Solar_Panel_Fit (Autodesk Fusion 360 design; units mm, degrees)
part number: 2026-09-24-14-30-26-043
Autodesk Fusion 360 part; units mm, degrees
sketch "Sketch1" plane through (0, 0, 0) normal (0, 0, 1) x (1, 0, 0)
  line L0 (0, 0) -> (145, 0)
  line L1 (145, 0) -> (145, -145)
  line L2 (145, -145) -> (0, -145)
  line L3 (0, -145) -> (0, 0)
  dimension "d1" = 145
  dimension "d2" = 145
  constraint horizontal L0
  constraint vertical L1
  constraint horizontal L2
  constraint vertical L3
  constraint coincident L0.start L3.end
  measures "d1" distance of L0.start L0.end
  measures "d2" distance of L0.start L2.end
extrude "Extrude1" add sketch "Sketch1" along normal blind 5 makes body 1
sketch "Sketch2" plane through (0, 0, 5) normal (0, 0, 1) x (-1, 0, 0)
  line L0 (0, 145) -> (-145, 145)
  line L1 (-145, 145) -> (-145, 0)
  line L2 (-145, 0) -> (0, 0)
  line L3 (0, 0) -> (0, 145)
  line L4 (-145, 145) -> (0, 145)
  line L5 (0, 145) -> (0, 0)
  line L6 (0, 0) -> (-145, 0)
  line L7 (-145, 0) -> (-145, 145)
  constraint horizontal L4
  constraint vertical L5
  constraint horizontal L6
  constraint vertical L7
  constraint coincident L2.end L3.start
  constraint coincident L0.end L1.start
extrude "Extrude2" add 1 faces at (48.3333, 0, 3.3333) along direction (0, 1, 0) blind 5 on bodies 1 bodies 1
extrude "Extrude3" add 1 faces at (145, -45, 1.6667) along direction (1, 0, 0) blind 5 on bodies 1 bodies 1
extrude "Extrude4" add 1 faces at (100, -145, 3.3333) along direction (0, -1, 0) blind 5 on bodies 1 bodies 1
extrude "Extrude5" add 1 faces at (0, -46.6667, 1.6667) along direction (-1, 0, 0) blind 5 on bodies 1 bodies 1
extrude "Extrude6" add sketch "Sketch2" along normal blind 5 bodies 1
extrude "Extrude7" add 1 faces at (96.6667, -96.6667, 10) along direction (0, 0, 1) blind 1 on bodies 1 bodies 1
extrude "Extrude8" add 1 faces at (96.6667, 3.3333, 5) along direction (0, 0, 1) blind 5 on bodies 1 bodies 1
extrude "Extrude9" cut 1 faces at (96.6667, -96.6667, 11) along direction (0, 0, -1) blind 6 on bodies 1 bodies 1
move_face "OffsetFaces1" offset -0.15 1 faces at (96.6667, 0, 6.6667) on bodies 1
extrude "Extrude10" cut 1 faces at (145, -96.6167, 8.3333) along direction (1, 0, 0) blind 0.15 on bodies 1 bodies 1
extrude "Extrude11" cut 1 faces at (48.3833, -145, 8.3333) along direction (0, -1, 0) blind 0.15 on bodies 1 bodies 1
extrude "Extrude12" cut 1 faces at (0, -48.2833, 8.3333) along direction (-1, 0, 0) blind 0.15 on bodies 1 bodies 1
extrude "Extrude13" add 1 faces at (46.6667, 5, 3.3333) along direction (0, 1, 0) blind 5 on bodies 1 bodies 1
extrude "Extrude14" add 1 faces at (-5, -43.3333, 3.3333) along direction (-1, 0, 0) blind 5 on bodies 1 bodies 1
extrude "Extrude15" add 1 faces at (150, -43.3333, 3.3333) along direction (1, 0, 0) blind 5 on bodies 1 bodies 1
extrude "Extrude16" add 1 faces at (100, -150, 3.3333) along direction (0, -1, 0) blind 5 on bodies 1 bodies 1
sketch "Sketch3" plane through (0, 0, 10) normal (0, 0, 1) x (-1, 0, 0)
  line L0 (0.15, -0.15) -> (-145.15, -0.15)
  line L1 (-145.15, -0.15) -> (-145.15, 145.15)
  line L2 (-145.15, 145.15) -> (0.15, 145.15)
  line L3 (0.15, 145.15) -> (0.15, -0.15)
  line L4 (-155, -10) -> (10, -10)
  line L5 (10, -10) -> (10, 155)
  line L6 (10, 155) -> (-155, 155)
  line L7 (-155, 155) -> (-155, -10)
  line L8 (10, -10) -> (10, 72.5) construction
  line L9 (10, 72.5) -> (0.15, 72.5) construction
  line L10 (0.15, 72.5) -> (0.15, 57.5) construction
  line L11 (0.15, 72.5) -> (0.15, 87.5) construction
  line L12 (0.15, 72.5) -> (0.15, 67.5) construction
  line L13 (0.15, 72.5) -> (0.15, 77.5) construction
  line L14 (0.15, 77.5) -> (10, 77.5) construction
  line L15 (10, 77.5) -> (5.075, 77.5) construction
  line L16 (0.15, 57.5) -> (5.075, 57.5) construction
  line L17 (0.15, 57.5) -> (2.6125, 57.5) construction
  line L18 (2.5, 57.5) -> (5.075, 57.5)
  line L19 (5.075, 57.5) -> (5.075, 87.5)
  line L20 (5.075, 87.5) -> (2.5, 87.5)
  line L21 (2.5, 87.5) -> (2.5, 57.5)
  dimension "d36" = 15
  dimension "d37" = 15
  dimension "d38" = 5
  dimension "d39" = 5
  dimension "d40" = 4.925
  constraint coincident L4.end L5.start
  constraint midpoint L5 L8.end
  constraint midpoint L3 L9.end
  constraint perpendicular L9 L10
  constraint perpendicular L9 L11
  constraint perpendicular L9 L12
  constraint perpendicular L9 L13
  constraint coincident L5 L14.end
  constraint perpendicular L5 L14
  constraint midpoint L14 L15.end
  constraint horizontal L16
  constraint midpoint L16 L17.end
  constraint horizontal L18
  constraint vertical L19
  constraint horizontal L20
  constraint vertical L21
  constraint coincident L16 L18.start
  measures "d36" distance of L9.end L10.end
  measures "d37" distance of L9.end L11.end
  measures "d38" distance of L9.end L12.end
  measures "d39" distance of L9.end L13.end
  measures "d40" distance of L10.end L16.end
extrude "Extrude17" cut sketch "Sketch3" against normal blind 5 contours L18 L19 L20 L21 bodies 1
sketch "Sketch4" plane through (0, 0, 10) normal (0, 0, 1) x (-1, 0, 0)
  line L0 (5.075, 57.5) -> (2.5, 57.5)
  line L1 (2.5, 57.5) -> (2.5, 87.5)
  line L2 (2.5, 87.5) -> (5.075, 87.5)
  line L3 (5.075, 87.5) -> (5.075, 57.5)
  line L4 (0.15, -0.15) -> (-145.15, -0.15)
  line L5 (-145.15, -0.15) -> (-145.15, 145.15)
  line L6 (-145.15, 145.15) -> (0.15, 145.15)
  line L7 (0.15, 145.15) -> (0.15, -0.15)
  line L8 (-155, -10) -> (10, -10)
  line L9 (10, -10) -> (10, 155)
  line L10 (10, 155) -> (-155, 155)
  line L11 (-155, 155) -> (-155, -10)
  line L12 (2.5, 57.5) -> (2.5, 87.5) construction
  line L13 (2.5, 87.5) -> (2.5, 72.5) construction
  line L14 (2.5, 72.5) -> (2.5, 80) construction
  line L15 (2.5, 72.5) -> (2.5, 57.5) construction
  line L16 (2.5, 57.5) -> (2.5, 65) construction
  line L17 (2.5, 65.1) -> (2.5, 80)
  line L18 (2.5, 80) -> (0.15, 80)
  line L19 (0.15, 80) -> (0.15, 65)
  line L20 (0.15, 65) -> (2.5, 65)
  line L21 (2.5, 65) -> (2.5, 80)
  constraint coincident L0.end L1.start
  constraint coincident L1.end L2.start
  constraint midpoint L12 L13.end
  constraint midpoint L13 L14.end
  constraint midpoint L15 L16.end
  constraint coincident L15 L17.start
  constraint horizontal L18
  constraint vertical L19
  constraint horizontal L20
  constraint vertical L21
  constraint coincident L7 L19.end
extrude "Extrude18" cut sketch "Sketch4" against normal blind 5 contours L1 L7 L17 L18 L19 L20 L21 bodies 1
sketch "Sketch5" plane through (0, 0, 10) normal (0, 0, 1) x (-1, 0, 0)
  line L0 (-155, -10) -> (10, -10)
  line L1 (10, -10) -> (10, 155)
  line L2 (10, 155) -> (-155, 155)
  line L3 (-155, 155) -> (-155, -10)
  line L4 (0.15, 80) -> (2.5, 80)
  line L5 (2.5, 80) -> (2.5, 87.5)
  line L6 (2.5, 87.5) -> (5.075, 87.5)
  line L7 (5.075, 87.5) -> (5.075, 57.5)
  line L8 (5.075, 57.5) -> (2.5, 57.5)
  line L9 (2.5, 57.5) -> (2.5, 65)
  line L10 (2.5, 65) -> (0.15, 65)
  line L11 (0.15, 65) -> (0.15, -0.15)
  line L12 (0.15, -0.15) -> (-145.15, -0.15)
  line L13 (-145.15, -0.15) -> (-145.15, 145.15)
  line L14 (-145.15, 145.15) -> (0.15, 145.15)
  line L15 (0.15, 145.15) -> (0.15, 80)
  line L16 (2.5, 57.5) -> (2.5, 65)
  line L17 (2.5, 65) -> (0.15, 65)
  line L18 (5.075, 57.5) -> (2.5, 57.5)
  line L19 (5.075, 87.5) -> (5.075, 57.5)
  line L20 (2.5, 87.5) -> (5.075, 87.5)
  line L21 (0.15, 80) -> (2.5, 80)
  line L22 (2.5, 80) -> (2.5, 87.5)
  line L23 (0.15, 80) -> (0.15, 65)
  line L24 (5.075, 57.5) -> (2.5, 57.5)
  line L25 (2.5, 57.5) -> (2.5, 65)
  line L26 (2.5, 65) -> (0.15, 65)
  line L27 (5.075, 57.5) -> (5.075, 87.5)
  line L28 (2.5, 87.5) -> (5.075, 87.5)
  line L29 (2.5, 87.5) -> (2.5, 80)
  line L30 (2.5, 80) -> (0.15, 80)
  line L31 (0.15, 80) -> (0.15, 65)
  constraint coincident L4.start L15.end
  constraint coincident L10.end L11.start
  constraint coincident L7.end L8.start
  constraint coincident L8.end L9.start
  constraint coincident L9.end L10.start
  constraint coincident L6.end L7.start
  constraint coincident L5.end L6.start
  constraint coincident L4.end L5.start
  constraint perpendicular L15 L30
extrude "Extrude19" add sketch "Sketch5" along normal blind 1 separate body contours L4 L5 L6 L7 L8 L9 L10 L16 L17 L18 L19 L20 L21 L22 L23 L24 L25 L26 L27 L28 L29 L30 L31 makes body 2
move_body "Move1" bodies 2 to x (-1, 0, 0) y (0, -1, 0) z (0, 0, 1) at (144.775, -145, 0)
copy_body "CopyPasteBodies1" bodies 2 makes body 3
move_body "Move2" bodies 3 to x (0, 1, 0) y (-1, 0, 0) z (0, 0, 1) at (-0.1125, -144.8875, 0)
copy_body "CopyPasteBodies2" bodies 3 makes body 4
move_body "Move3" bodies 4 to x (-1, 0, 0) y (0, -1, 0) z (0, 0, 1) at (144.775, -145, 0)
extrude "Extrude20" cut 3 faces at (148.9917, -75, 11) (74.8875, -149.1042, 11) (74.8875, 4.1042, 11) along direction (0, 0, -1) blind 6 on bodies 2 3 4 bodies 1 2 3 4
extrude "Extrude21" cut 1 faces at (148.1333, -57.5, 8.3333) along direction (0, 1, 0) blind 5 on bodies 1 bodies 1
extrude "Extrude22" cut 1 faces at (148.9917, -87.5, 8.3333) along direction (0, -1, 0) blind 5 on bodies 1 bodies 1
extrude "Extrude23" cut 1 faces at (87.3875, 4.1042, 8.3333) along direction (1, 0, 0) blind 5 on bodies 1 bodies 1
extrude "Extrude24" cut 1 faces at (57.3875, 3.2458, 8.3333) along direction (-1, 0, 0) blind 5 on bodies 1 bodies 1
extrude "Extrude25" cut 1 faces at (-4.2167, -87.5, 8.3333) along direction (0, -1, 0) blind 5 on bodies 1 bodies 1
extrude "Extrude26" cut 1 faces at (-3.3583, -57.5, 8.3333) along direction (0, 1, 0) blind 5 on bodies 1 bodies 1
extrude "Extrude27" cut 1 faces at (57.3875, -149.1042, 8.3333) along direction (-1, 0, 0) blind 5 on bodies 1 bodies 1
extrude "Extrude28" cut 1 faces at (87.3875, -148.2458, 8.3333) along direction (1, 0, 0) blind 5 on bodies 1 bodies 1
extrude "Extrude29" cut 1 faces at (52.3875, -149.1042, 8.3333) along direction (-1, 0, 0) blind 2.5 on bodies 1 bodies 1
extrude "Extrude30" cut 1 faces at (92.3875, -148.2458, 8.3333) along direction (1, 0, 0) blind 2.5 on bodies 1 bodies 1
extrude "Extrude31" cut 1 faces at (-4.2167, -92.5, 8.3333) along direction (0, -1, 0) blind 2.5 on bodies 1 bodies 1
extrude "Extrude32" cut 1 faces at (-3.3583, -52.5, 8.3333) along direction (0, 1, 0) blind 2.5 on bodies 1 bodies 1
extrude "Extrude33" cut 1 faces at (52.3875, 3.2458, 8.3333) along direction (-1, 0, 0) blind 2.5 on bodies 1 bodies 1
extrude "Extrude34" cut 1 faces at (92.3875, 4.1042, 8.3333) along direction (1, 0, 0) blind 2.5 on bodies 1 bodies 1
extrude "Extrude35" cut 1 faces at (148.1333, -52.5, 8.3333) along direction (0, 1, 0) blind 2.5 on bodies 1 bodies 1
extrude "Extrude36" cut 1 faces at (148.9917, -92.5, 8.3333) along direction (0, -1, 0) blind 2.5 on bodies 1 bodies 1
extrude "Extrude37" add 1 faces at (53.2083, -70, 5) along direction (0, 0, 1) blind 2.5 on bodies 1 bodies 1 2 3 4
sketch "Sketch6" plane through (0, 0, 10) normal (0, 0, 1) x (-1, 0, 0)
  line L0 (-149.85, 50) -> (-149.85, 95)
  line L1 (-149.85, 95) -> (-147.275, 95)
  line L2 (-147.275, 95) -> (-147.275, 80)
  line L3 (-147.275, 80) -> (-145.15, 80)
  line L4 (-145.15, 80) -> (-145.15, 145.15)
  line L5 (-145.15, 145.15) -> (-79.8875, 145.15)
  line L6 (-79.8875, 145.15) -> (-79.8875, 147.3875)
  line L7 (-79.8875, 147.3875) -> (-94.8875, 147.3875)
  line L8 (-94.8875, 147.3875) -> (-94.8875, 149.9625)
  line L9 (-94.8875, 149.9625) -> (-49.8875, 149.9625)
  line L10 (-49.8875, 149.9625) -> (-49.8875, 147.3875)
  line L11 (-49.8875, 147.3875) -> (-64.8875, 147.3875)
  line L12 (-64.8875, 147.3875) -> (-64.8875, 145.15)
  line L13 (-64.8875, 145.15) -> (0.15, 145.15)
  line L14 (0.15, 145.15) -> (0.15, 80)
  line L15 (0.15, 80) -> (2.5, 80)
  line L16 (2.5, 80) -> (2.5, 95)
  line L17 (2.5, 95) -> (5.075, 95)
  line L18 (5.075, 95) -> (5.075, 50)
  line L19 (5.075, 50) -> (2.5, 50)
  line L20 (2.5, 50) -> (2.5, 65)
  line L21 (2.5, 65) -> (0.15, 65)
  line L22 (0.15, 65) -> (0.15, -0.15)
  line L23 (0.15, -0.15) -> (-64.8875, -0.15)
  line L24 (-64.8875, -0.15) -> (-64.8875, -2.3875)
  line L25 (-64.8875, -2.3875) -> (-49.8875, -2.3875)
  line L26 (-49.8875, -2.3875) -> (-49.8875, -4.9625)
  line L27 (-49.8875, -4.9625) -> (-94.8875, -4.9625)
  line L28 (-94.8875, -4.9625) -> (-94.8875, -2.3875)
  line L29 (-94.8875, -2.3875) -> (-79.8875, -2.3875)
  line L30 (-79.8875, -2.3875) -> (-79.8875, -0.15)
  line L31 (-79.8875, -0.15) -> (-145.15, -0.15)
  line L32 (-145.15, -0.15) -> (-145.15, 65)
  line L33 (-145.15, 65) -> (-147.275, 65)
  line L34 (-147.275, 65) -> (-147.275, 50)
  line L35 (-147.275, 50) -> (-149.85, 50)
  line L36 (-155, -10) -> (10, -10)
  line L37 (10, -10) -> (10, 155)
  line L38 (10, 155) -> (-155, 155)
  line L39 (-155, 155) -> (-155, -10)
  line L40 (0.15, 145.15) -> (0.15, 95) construction
  line L41 (0.15, 95) -> (0.15, 120.075) construction
  circle A0 centre (0.15, 120.075) radius 5
  dimension "d83" = 10
  constraint coincident L13.end L14.start
  constraint coincident L14 L40.end
  constraint midpoint L40 L41.end
  constraint coincident L41.end A0.centre
  measures "d83" diameter of A0
extrude "Extrude38" cut sketch "Sketch6" against normal blind 2.5 contours L14 A0 picked at (1.5521, 119.1739) bodies 1
extrude "Extrude39" add 1 faces at (100, -45, 0) along direction (0, 0, -1) blind 5 on bodies 1 bodies 1
move_body "Move4" bodies 1 to x (1, 0, 0) y (0, 1, 0) z (0, 0, 1) at (0, 0, 5)
sketch "Sketch7" plane through (0, 0, 12.5) normal (0, 0, 1) x (-1, 0, 0)
  line L0 (-79.8875, 145.15) -> (-145.15, 145.15)
  line L1 (-145.15, 145.15) -> (-145.15, 80)
  line L2 (-145.15, 80) -> (-147.275, 80)
  line L3 (-147.275, 80) -> (-147.275, 95)
  line L4 (-147.275, 95) -> (-149.85, 95)
  line L5 (-149.85, 95) -> (-149.85, 50)
  line L6 (-149.85, 50) -> (-147.275, 50)
  line L7 (-147.275, 50) -> (-147.275, 65)
  line L8 (-147.275, 65) -> (-145.15, 65)
  line L9 (-145.15, 65) -> (-145.15, -0.15)
  line L10 (-145.15, -0.15) -> (-79.8875, -0.15)
  line L11 (-79.8875, -0.15) -> (-79.8875, -2.3875)
  line L12 (-79.8875, -2.3875) -> (-94.8875, -2.3875)
  line L13 (-94.8875, -2.3875) -> (-94.8875, -4.9625)
  line L14 (-94.8875, -4.9625) -> (-49.8875, -4.9625)
  line L15 (-49.8875, -4.9625) -> (-49.8875, -2.3875)
  line L16 (-49.8875, -2.3875) -> (-64.8875, -2.3875)
  line L17 (-64.8875, -2.3875) -> (-64.8875, -0.15)
  line L18 (-64.8875, -0.15) -> (0.15, -0.15)
  line L19 (0.15, -0.15) -> (0.15, 65)
  line L20 (0.15, 65) -> (2.5, 65)
  line L21 (2.5, 65) -> (2.5, 50)
  line L22 (2.5, 50) -> (5.075, 50)
  line L23 (5.075, 50) -> (5.075, 95)
  line L24 (5.075, 95) -> (2.5, 95)
  line L25 (2.5, 95) -> (2.5, 80)
  line L26 (2.5, 80) -> (0.15, 80)
  line L27 (0.15, 80) -> (0.15, 115.075)
  arc A0 (0.15, 115.075) -> (0.15, 125.075) centre (0.15, 120.075) ccw
  line L28 (0.15, 125.075) -> (0.15, 145.15)
  line L29 (0.15, 145.15) -> (-64.8875, 145.15)
  line L30 (-64.8875, 145.15) -> (-64.8875, 147.3875)
  line L31 (-64.8875, 147.3875) -> (-49.8875, 147.3875)
  line L32 (-49.8875, 147.3875) -> (-49.8875, 149.9625)
  line L33 (-49.8875, 149.9625) -> (-94.8875, 149.9625)
  line L34 (-94.8875, 149.9625) -> (-94.8875, 147.3875)
  line L35 (-94.8875, 147.3875) -> (-79.8875, 147.3875)
  line L36 (-79.8875, 147.3875) -> (-79.8875, 145.15)
  line L37 (10, 155) -> (-155, 155) construction
  line L38 (-155, 155) -> (-72.5, 155) construction
  line L39 (-72.5, 155) -> (-72.3875, 149.9625) construction
  line L40 (-72.3875, 149.9625) -> (-72.3875, 137.4625) construction
  line L41 (-72.3875, 137.4625) -> (-97.3875, 137.4625) construction
  line L42 (-72.3875, 137.4625) -> (-47.3875, 137.4625) construction
  line L43 (-72.3875, 137.4625) -> (-72.3875, 92.4625) construction
  line L44 (-72.3875, 92.4625) -> (-47.3875, 92.4625) construction
  line L45 (-47.3875, 92.4625) -> (-97.3875, 92.4625)
  line L46 (-97.3875, 92.4625) -> (-97.3875, 137.4625)
  line L47 (-97.3875, 137.4625) -> (-47.3875, 137.4625)
  line L48 (-47.3875, 137.4625) -> (-47.3875, 92.4625)
  dimension "d88" = 12.5
  dimension "d89" = 25
  dimension "d90" = 25
  dimension "d91" = 45
  constraint perpendicular L28 L37
  constraint midpoint L37 L38.end
  constraint midpoint L33 L39.end
  constraint perpendicular L33 L40
  constraint perpendicular L40 L41
  constraint perpendicular L40 L42
  constraint perpendicular L42 L43
  constraint perpendicular L43 L44
  constraint horizontal L45
  constraint vertical L46
  constraint horizontal L47
  constraint vertical L48
  measures "d88" distance of L39.end L40.end
  measures "d89" distance of L40.end L41.end
  measures "d90" distance of L40.end L42.end
  measures "d91" distance of L40.end L43.end
extrude "Extrude40" cut sketch "Sketch7" against normal blind 70 contours L45 L46 L47 L48 bodies 1
sketch "Sketch8" plane through (0, 0, 12.5) normal (0, 0, 1) x (-1, 0, 0)
  line L0 (-97.3875, 92.4625) -> (-97.3875, 137.4625)
  line L1 (-97.3875, 137.4625) -> (-47.3875, 137.4625)
  line L2 (-47.3875, 137.4625) -> (-47.3875, 92.4625)
  line L3 (-47.3875, 92.4625) -> (-97.3875, 92.4625)
  line L4 (-79.8875, 145.15) -> (-145.15, 145.15)
  line L5 (-145.15, 145.15) -> (-145.15, 80)
  line L6 (-145.15, 80) -> (-147.275, 80)
  line L7 (-147.275, 80) -> (-147.275, 95)
  line L8 (-147.275, 95) -> (-149.85, 95)
  line L9 (-149.85, 95) -> (-149.85, 50)
  line L10 (-149.85, 50) -> (-147.275, 50)
  line L11 (-147.275, 50) -> (-147.275, 65)
  line L12 (-147.275, 65) -> (-145.15, 65)
  line L13 (-145.15, 65) -> (-145.15, -0.15)
  line L14 (-145.15, -0.15) -> (-79.8875, -0.15)
  line L15 (-79.8875, -0.15) -> (-79.8875, -2.3875)
  line L16 (-79.8875, -2.3875) -> (-94.8875, -2.3875)
  line L17 (-94.8875, -2.3875) -> (-94.8875, -4.9625)
  line L18 (-94.8875, -4.9625) -> (-49.8875, -4.9625)
  line L19 (-49.8875, -4.9625) -> (-49.8875, -2.3875)
  line L20 (-49.8875, -2.3875) -> (-64.8875, -2.3875)
  line L21 (-64.8875, -2.3875) -> (-64.8875, -0.15)
  line L22 (-64.8875, -0.15) -> (0.15, -0.15)
  line L23 (0.15, -0.15) -> (0.15, 65)
  line L24 (0.15, 65) -> (2.5, 65)
  line L25 (2.5, 65) -> (2.5, 50)
  line L26 (2.5, 50) -> (5.075, 50)
  line L27 (5.075, 50) -> (5.075, 95)
  line L28 (5.075, 95) -> (2.5, 95)
  line L29 (2.5, 95) -> (2.5, 80)
  line L30 (2.5, 80) -> (0.15, 80)
  line L31 (0.15, 80) -> (0.15, 115.075)
  arc A0 (0.15, 115.075) -> (0.15, 125.075) centre (0.15, 120.075) ccw
  line L32 (0.15, 125.075) -> (0.15, 145.15)
  line L33 (0.15, 145.15) -> (-64.8875, 145.15)
  line L34 (-64.8875, 145.15) -> (-64.8875, 147.3875)
  line L35 (-64.8875, 147.3875) -> (-49.8875, 147.3875)
  line L36 (-49.8875, 147.3875) -> (-49.8875, 149.9625)
  line L37 (-49.8875, 149.9625) -> (-94.8875, 149.9625)
  line L38 (-94.8875, 149.9625) -> (-94.8875, 147.3875)
  line L39 (-94.8875, 147.3875) -> (-79.8875, 147.3875)
  line L40 (-79.8875, 147.3875) -> (-79.8875, 145.15)
  line L41 (-97.3875, 92.4625) -> (-47.3875, 92.4625) construction
  line L42 (-47.3875, 92.4625) -> (-72.3875, 92.4625) construction
  circle A1 centre (-72.3875, 92.4625) radius 10
  dimension "d94" = 20
  constraint coincident L0.start L3.end
  constraint coincident L2.end L3.start
  constraint midpoint L41 L42.end
  constraint coincident L42.end A1.centre
  measures "d94" diameter of A1
extrude "Extrude41" cut sketch "Sketch8" against normal blind 28 contours L3 A1 picked at (-74.6478, 87.4276) bodies 1
sketch "Sketch9" plane through (0, 0, 12.5) normal (0, 0, 1) x (-1, 0, 0)
  line L0 (-79.8875, 145.15) -> (-145.15, 145.15)
  line L1 (-145.15, 145.15) -> (-145.15, 80)
  line L2 (-145.15, 80) -> (-147.275, 80)
  line L3 (-147.275, 80) -> (-147.275, 95)
  line L4 (-147.275, 95) -> (-149.85, 95)
  line L5 (-149.85, 95) -> (-149.85, 50)
  line L6 (-149.85, 50) -> (-147.275, 50)
  line L7 (-147.275, 50) -> (-147.275, 65)
  line L8 (-147.275, 65) -> (-145.15, 65)
  line L9 (-145.15, 65) -> (-145.15, -0.15)
  line L10 (-145.15, -0.15) -> (-79.8875, -0.15)
  line L11 (-79.8875, -0.15) -> (-79.8875, -2.3875)
  line L12 (-79.8875, -2.3875) -> (-94.8875, -2.3875)
  line L13 (-94.8875, -2.3875) -> (-94.8875, -4.9625)
  line L14 (-94.8875, -4.9625) -> (-49.8875, -4.9625)
  line L15 (-49.8875, -4.9625) -> (-49.8875, -2.3875)
  line L16 (-49.8875, -2.3875) -> (-64.8875, -2.3875)
  line L17 (-64.8875, -2.3875) -> (-64.8875, -0.15)
  line L18 (-64.8875, -0.15) -> (0.15, -0.15)
  line L19 (0.15, -0.15) -> (0.15, 65)
  line L20 (0.15, 65) -> (2.5, 65)
  line L21 (2.5, 65) -> (2.5, 50)
  line L22 (2.5, 50) -> (5.075, 50)
  line L23 (5.075, 50) -> (5.075, 95)
  line L24 (5.075, 95) -> (2.5, 95)
  line L25 (2.5, 95) -> (2.5, 80)
  line L26 (2.5, 80) -> (0.15, 80)
  line L27 (0.15, 80) -> (0.15, 115.075)
  arc A0 (0.15, 115.075) -> (0.15, 125.075) centre (0.15, 120.075) ccw
  line L28 (0.15, 125.075) -> (0.15, 145.15)
  line L29 (0.15, 145.15) -> (-64.8875, 145.15)
  line L30 (-64.8875, 145.15) -> (-64.8875, 147.3875)
  line L31 (-64.8875, 147.3875) -> (-49.8875, 147.3875)
  line L32 (-49.8875, 147.3875) -> (-49.8875, 149.9625)
  line L33 (-49.8875, 149.9625) -> (-94.8875, 149.9625)
  line L34 (-94.8875, 149.9625) -> (-94.8875, 147.3875)
  line L35 (-94.8875, 147.3875) -> (-79.8875, 147.3875)
  line L36 (-79.8875, 147.3875) -> (-79.8875, 145.15)
  arc A1 (-82.3875, 92.4625) -> (-62.3875, 92.4625) centre (-72.3875, 92.4625) ccw
  line L37 (-82.3875, 92.4625) -> (-97.3875, 92.4625)
  line L38 (-97.3875, 92.4625) -> (-97.3875, 137.4625)
  line L39 (-97.3875, 137.4625) -> (-47.3875, 137.4625)
  line L40 (-47.3875, 137.4625) -> (-47.3875, 92.4625)
  line L41 (-47.3875, 92.4625) -> (-62.3875, 92.4625)
  circle A2 centre (0.15, 120.075) radius 7.5
  dimension "d97" = 15
  constraint concentric A0 A2
  measures "d97" diameter of A2
sketch "Sketch10" plane through (0, 0, 15) normal (0, 0, 1) x (-1, 0, 0)
  line L0 (-155, -10) -> (10, -10)
  line L1 (10, -10) -> (10, 155)
  line L2 (10, 155) -> (-155, 155)
  line L3 (-155, 155) -> (-155, -10)
  arc A0 (0.15, 115.075) -> (0.15, 125.075) centre (0.15, 120.075) ccw
  line L4 (0.15, 115.075) -> (0.15, 80)
  line L5 (0.15, 80) -> (2.5, 80)
  line L6 (2.5, 80) -> (2.5, 95)
  line L7 (2.5, 95) -> (5.075, 95)
  line L8 (5.075, 95) -> (5.075, 50)
  line L9 (5.075, 50) -> (2.5, 50)
  line L10 (2.5, 50) -> (2.5, 65)
  line L11 (2.5, 65) -> (0.15, 65)
  line L12 (0.15, 65) -> (0.15, -0.15)
  line L13 (0.15, -0.15) -> (-64.8875, -0.15)
  line L14 (-64.8875, -0.15) -> (-64.8875, -2.3875)
  line L15 (-64.8875, -2.3875) -> (-49.8875, -2.3875)
  line L16 (-49.8875, -2.3875) -> (-49.8875, -4.9625)
  line L17 (-49.8875, -4.9625) -> (-94.8875, -4.9625)
  line L18 (-94.8875, -4.9625) -> (-94.8875, -2.3875)
  line L19 (-94.8875, -2.3875) -> (-79.8875, -2.3875)
  line L20 (-79.8875, -2.3875) -> (-79.8875, -0.15)
  line L21 (-79.8875, -0.15) -> (-145.15, -0.15)
  line L22 (-145.15, -0.15) -> (-145.15, 65)
  line L23 (-145.15, 65) -> (-147.275, 65)
  line L24 (-147.275, 65) -> (-147.275, 50)
  line L25 (-147.275, 50) -> (-149.85, 50)
  line L26 (-149.85, 50) -> (-149.85, 95)
  line L27 (-149.85, 95) -> (-147.275, 95)
  line L28 (-147.275, 95) -> (-147.275, 80)
  line L29 (-147.275, 80) -> (-145.15, 80)
  line L30 (-145.15, 80) -> (-145.15, 145.15)
  line L31 (-145.15, 145.15) -> (-79.8875, 145.15)
  line L32 (-79.8875, 145.15) -> (-79.8875, 147.3875)
  line L33 (-79.8875, 147.3875) -> (-94.8875, 147.3875)
  line L34 (-94.8875, 147.3875) -> (-94.8875, 149.9625)
  line L35 (-94.8875, 149.9625) -> (-49.8875, 149.9625)
  line L36 (-49.8875, 149.9625) -> (-49.8875, 147.3875)
  line L37 (-49.8875, 147.3875) -> (-64.8875, 147.3875)
  line L38 (-64.8875, 147.3875) -> (-64.8875, 145.15)
  line L39 (-64.8875, 145.15) -> (0.15, 145.15)
  line L40 (0.15, 145.15) -> (0.15, 125.075)
  circle A1 centre (0.15, 120.075) radius 7.5
  dimension "d98" = 15
  constraint concentric A0 A1
  measures "d98" diameter of A1
extrude "Extrude42" cut sketch "Sketch10" against normal blind 2 contours A0 L4 L40 A1 picked at (6.7866, 119.5947) bodies 1
extrude "Extrude43" cut 1 faces at (-0.5226, -113.4363, 13) along direction (0, 0, -1) blind 0.5 on bodies 1 bodies 1
